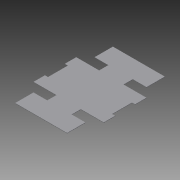
# Autodesk Inventor part: polycarb base
Saved by Autodesk Inventor 2015 SP1 (Build 190203100, 203)
## iProperties
Created: 2015-01-13
Part Number: polycarb base
Material: Generic
Document SubType Name: Modeling
Designer: Jarod
Density: 1 g/cm^3
Appearance: Default
Author: Jarod
Autodesk Inventor part; units mm, degrees
ref_plane "YZ Plane" through (0, 0, 0) normal (1, 0, 0) x (0, 1, 0)
ref_plane "XZ Plane" through (0, 0, 0) normal (0, 1, 0) x (-1, 0, 0)
ref_plane "XY Plane" through (0, 0, 0) normal (0, 0, 1) x (1, 0, 0)
sketch "Sketch1" plane through (0, 0, 0) normal (0, 1, 0) x (-1, 0, 0)
  line L0 (0, 0) -> (-584.2, 0)
  line L1 (-584.2, 0) -> (-584.2, -812.8)
  line L2 (-584.2, -812.8) -> (0, -812.8)
  line L3 (0, -812.8) -> (0, 0)
  dimension "d0" = 584.2
  dimension "d1" = 812.8
  constraints: 8 end point, 2 parallel, 1 horizontal, 1 perpendicular
  measures "d0" distance of L2.end L1.end
  measures "d1" distance of L1.end L0.end
extrude "Extrusion1" add sketch "Sketch1" along normal blind 3.175
sketch "Sketch2" plane through (0, 0, 0) normal (0, -1, 0) x (1, 0, 0)
  line L0 (0, 0) -> (584.2, 0) projected
  line L1 (0, -812.8) -> (0, 0) projected
  line L2 (584.2, -812.8) -> (0, -812.8) projected
  line L3 (584.2, 0) -> (584.2, -812.8) projected
  line L4 (584.2, 0) -> (584.2, -812.8) projected
  line L5 (584.2, -323.85) -> (558.8, -323.85)
  line L6 (558.8, -323.85) -> (558.8, -488.95)
  line L7 (558.8, -488.95) -> (584.2, -488.95)
  line L8 (584.2, -488.95) -> (584.2, -323.85)
  line L9 (0, -812.8) -> (0, 0) projected
  line L10 (0, -323.85) -> (25.4, -323.85)
  line L11 (25.4, -323.85) -> (25.4, -488.95)
  line L12 (25.4, -488.95) -> (0, -488.95)
  line L13 (0, -488.95) -> (0, -323.85)
  line L14 (584.2, 0) -> (508, 0)
  line L15 (508, 0) -> (508, -228.6)
  line L16 (508, -228.6) -> (584.2, -228.6)
  line L17 (584.2, -228.6) -> (584.2, 0)
  line L18 (0, 0) -> (76.2, 0)
  line L19 (76.2, 0) -> (76.2, -228.6)
  line L20 (76.2, -228.6) -> (0, -228.6)
  line L21 (0, -228.6) -> (0, 0)
  line L22 (0, -812.8) -> (76.2, -812.8)
  line L23 (76.2, -812.8) -> (76.2, -584.2)
  line L24 (76.2, -584.2) -> (0, -584.2)
  line L25 (0, -584.2) -> (0, -812.8)
  line L26 (584.2, -812.8) -> (508, -812.8)
  line L27 (508, -812.8) -> (508, -584.2)
  line L28 (508, -584.2) -> (584.2, -584.2)
  line L29 (584.2, -584.2) -> (584.2, -812.8)
  line L30 (508, -228.6) -> (393.7, -228.6)
  line L31 (393.7, -228.6) -> (393.7, -152.4)
  line L32 (393.7, -152.4) -> (508, -152.4)
  line L33 (508, -152.4) -> (508, -228.6)
  line L34 (508, -584.2) -> (393.7, -584.2)
  line L35 (393.7, -584.2) -> (393.7, -660.4)
  line L36 (393.7, -660.4) -> (508, -660.4)
  line L37 (508, -660.4) -> (508, -584.2)
  line L38 (76.2, -584.2) -> (190.5, -584.2)
  line L39 (190.5, -584.2) -> (190.5, -660.4)
  line L40 (190.5, -660.4) -> (76.2, -660.4)
  line L41 (76.2, -660.4) -> (76.2, -584.2)
  line L42 (76.2, -228.6) -> (190.5, -228.6)
  line L43 (190.5, -228.6) -> (190.5, -152.4)
  line L44 (190.5, -152.4) -> (76.2, -152.4)
  line L45 (76.2, -152.4) -> (76.2, -228.6)
  dimension "d4" = 165.1
  dimension "d5" = 165.1
  dimension "d6" = 25.4
  dimension "d7" = 25.4
  dimension "d8" = 323.85
  dimension "d9" = 323.85
  dimension "d10" = 76.2
  dimension "d11" = 228.6
  dimension "d12" = 76.2
  dimension "d13" = 228.6
  dimension "d14" = 76.2
  dimension "d15" = 228.6
  dimension "d16" = 76.2
  dimension "d17" = 228.6
  dimension "d18" = 114.3
  dimension "d19" = 76.2
  dimension "d20" = 114.3
  dimension "d21" = 76.2
  dimension "d22" = 114.3
  dimension "d23" = 76.2
  dimension "d24" = 114.3
  dimension "d25" = 76.2
  constraints: 80 end point, 20 parallel, 10 horizontal, 10 perpendicular, 2 point on line
  measures "d4" distance between parallel lines of L7 L5
  measures "d5" distance between parallel lines of L12 L10
  measures "d6" distance between parallel lines of L8 L6
  measures "d7" distance between parallel lines of L1 L11
  measures "d8" distance between parallel lines of L0 L10
  measures "d9" distance between parallel lines of L0 L5
  measures "d10" distance of L16.end L15.end
  measures "d11" distance of L15.end L14.end
  measures "d12" distance of L19.end L20.end
  measures "d13" distance of L18.end L19.end
  measures "d14" distance of L24.end L23.end
  measures "d15" distance of L23.end L22.end
  measures "d16" distance of L27.end L28.end
  measures "d17" distance of L26.end L27.end
  measures "d18" distance of L31.end L32.end
  measures "d19" distance of L30.end L31.end
  measures "d20" distance of L36.end L35.end
  measures "d21" distance of L35.end L34.end
  measures "d22" distance of L39.end L40.end
  measures "d23" distance of L38.end L39.end
  measures "d24" distance of L44.end L43.end
  measures "d25" distance of L43.end L42.end
extrude "Extrusion2" cut sketch "Sketch2" against normal blind 3.175 contours L0 L19 L20 L1 | L0 L3 L16 L15 | L44 L43 L42 L19 | L10 L11 L12 L1 | L15 L30 L31 L32 | L24 L23 L2 L1 | L3 L7 L6 L5 | L38 L39 L40 L23 | L3 L2 L27 L28 | L27 L36 L35 L34
body "Solid1"
